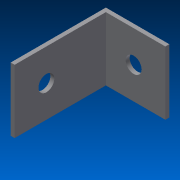
# Autodesk Inventor part: LBrace
Saved by Autodesk Inventor 2013 (Build 170138000, 138)
## iProperties
Created: 2013-07-23
Part Number: LBrace
Material: Aluminum 6061
Document SubType Name: Modeling
Designer: orange
Density: 1 g/cm^3
Author: orange
Autodesk Inventor part; units mm, degrees
ref_plane "YZ Plane" through (0, 0, 0) normal (1, 0, 0) x (0, 1, 0)
ref_plane "XZ Plane" through (0, 0, 0) normal (0, 1, 0) x (-1, 0, 0)
ref_plane "XY Plane" through (0, 0, 0) normal (0, 0, 1) x (1, 0, 0)
sketch "Sketch1" plane through (0, 0, 0) normal (1, 0, 0) x (0, 1, 0)
  line L0 (0, 0) -> (25.4, 0)
  line L1 (25.4, 0) -> (25.4, 38.1)
  line L2 (25.4, 38.1) -> (0, 38.1)
  line L3 (0, 38.1) -> (0, 0)
  dimension "d0" = 25.4
  dimension "d1" = 38.1
  constraints: 8 end point, 2 parallel, 1 horizontal, 1 perpendicular
  measures "d0" distance of L0.start L0.end
  measures "d1" distance of L2.end L0.start
extrude "Extrusion1" add sketch "Sketch1" along normal blind 1.5875
sketch "Sketch2" plane through (1.5875, 0, 0) normal (1, 0, 0) x (0, 0, -1)
  line L0 (-38.1, 0) -> (0, 0) projected
  line L1 (0, 25.4) -> (-1.5875, 25.4)
  line L2 (-1.5875, 25.4) -> (-1.5875, 0)
  line L3 (-1.5875, 0) -> (0, 0)
  line L4 (0, 0) -> (0, 25.4)
  dimension "d4" = 1.5875
  constraints: 8 end point, 2 parallel, 1 horizontal, 1 perpendicular, 1 point on line
  measures "d4" distance between parallel lines of L4 L2
extrude "Extrusion2" add sketch "Sketch2" along normal blind 23.8125
sketch "Sketch3" plane through (1.5875, 0, 0) normal (1, 0, 0) x (0, 0, -1)
  line L0 (-1.5875, 25.4) -> (-38.1, 25.4) projected
  line L1 (-38.1, 25.4) -> (-38.1, 0) projected
  point P0 (0, 0)
  point P1 (-25.3973, 12.7)
  dimension "d8" = 12.7027
  dimension "d9" = 12.7
  measures "d8" distance from line of L1 point (-25.397, 12.7)
  measures "d9" distance from line of L0 point (-25.397, 12.7)
hole "Hole1" at (1.5875, 12.7, 25.3973) direction (-1, 0, 0) diameter 6.35 end through all
sketch "Sketch4" plane through (1.5875, 0, 1.5875) normal (0, 0, 1) x (1, 0, 0)
  line L0 (23.8125, 25.4) -> (23.8125, 0) projected
  line L1 (0, 25.4) -> (23.8125, 25.4) projected
  point P0 (-1.5875, 0)
  point P1 (11.1125, 12.7)
  dimension "d17" = 12.7
  dimension "d18" = 12.7
  measures "d17" distance from line of L0 point (11.113, 12.7)
  measures "d18" distance from line of point (11.113, 12.7) L1
hole "Hole2" at (12.7, 12.7, 1.5875) direction (0, 0, -1) diameter 6.35 end through all
body "Solid1"
